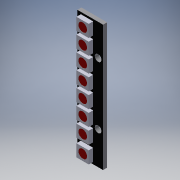
# Autodesk Inventor part: Neopixel_Stick
Saved by Autodesk Inventor 2016 (Build 200138000, 138)
## iProperties
Created: 2018-09-26
Part Number: Neopixel_Stick
Material: Generic
Document SubType Name: Modeling
Designer: Student
Density: 1 g/cm^3
Appearance: Default
Author: Student
Autodesk Inventor part; units mm, degrees
ref_plane "YZ Plane" through (0, 0, 0) normal (1, 0, 0) x (0, 1, 0)
ref_plane "XZ Plane" through (0, 0, 0) normal (0, 1, 0) x (-1, 0, 0)
ref_plane "XY Plane" through (0, 0, 0) normal (0, 0, 1) x (1, 0, 0)
sketch "Sketch1" plane through (0, 0, 0) normal (0, 0, 1) x (1, 0, 0)
  line L0 (0, 0) -> (10.414, 0)
  line L1 (10.414, 0) -> (10.414, 50.8)
  line L2 (10.414, 50.8) -> (0, 50.8)
  line L3 (0, 50.8) -> (0, 0)
  dimension "d0" = 10.414
  dimension "d1" = 50.8
  constraints: 8 end point, 2 parallel, 1 horizontal, 1 perpendicular
  measures "d0" distance of L2.end L1.end
  measures "d1" distance of L1.end L0.end
extrude "Extrusion1" add sketch "Sketch1" along normal blind 1.651
sketch "Sketch2" plane through (0, 0, 1.651) normal (0, 0, 1) x (1, 0, 0)
  line L0 (0, 0) -> (10.414, 0) projected
  line L1 (5.207, 0) -> (3.937, 0)
  line L2 (3.937, 0) -> (3.937, 3.302)
  circle A0 centre (3.937, 3.302) radius 1.778
  line L3 (10.414, 50.8) -> (0, 50.8) projected
  line L4 (5.207, 50.8) -> (3.937, 50.8)
  line L5 (3.937, 50.8) -> (3.937, 47.498)
  circle A1 centre (3.937, 47.498) radius 1.778
  line L6 (3.937, 47.498) -> (3.937, 41.275)
  line L7 (3.937, 41.275) -> (3.937, 35.052)
  line L8 (3.937, 35.052) -> (3.937, 28.829)
  line L9 (3.937, 28.829) -> (3.937, 22.606)
  line L10 (3.937, 22.606) -> (3.937, 16.383)
  line L11 (3.937, 16.383) -> (3.937, 10.16)
  line L12 (3.937, 10.16) -> (3.937, 3.302)
  circle A2 centre (3.937, 10.16) radius 1.778
  circle A3 centre (3.937, 16.383) radius 1.778
  circle A4 centre (3.937, 22.606) radius 1.778
  circle A5 centre (3.937, 28.829) radius 1.778
  circle A6 centre (3.937, 35.052) radius 1.778
  circle A7 centre (3.937, 41.275) radius 1.778
  line L13 (1.4605, 45.0215) -> (6.4135, 45.0215)
  line L14 (6.4135, 45.0215) -> (6.4135, 49.9745)
  line L15 (6.4135, 49.9745) -> (1.4605, 49.9745)
  line L16 (1.4605, 49.9745) -> (1.4605, 45.0215)
  line L17 (1.4605, 45.0215) -> (6.4135, 49.9745) construction
  line L18 (6.4135, 45.0215) -> (1.4605, 49.9745) construction
  line L19 (1.4605, 38.7985) -> (6.4135, 38.7985)
  line L20 (6.4135, 38.7985) -> (6.4135, 43.7515)
  line L21 (6.4135, 43.7515) -> (1.4605, 43.7515)
  line L22 (1.4605, 43.7515) -> (1.4605, 38.7985)
  line L23 (1.4605, 38.7985) -> (6.4135, 43.7515) construction
  line L24 (6.4135, 38.7985) -> (1.4605, 43.7515) construction
  line L25 (1.4605, 32.5755) -> (6.4135, 32.5755)
  line L26 (6.4135, 32.5755) -> (6.4135, 37.5285)
  line L27 (6.4135, 37.5285) -> (1.4605, 37.5285)
  line L28 (1.4605, 37.5285) -> (1.4605, 32.5755)
  line L29 (1.4605, 32.5755) -> (6.4135, 37.5285) construction
  line L30 (6.4135, 32.5755) -> (1.4605, 37.5285) construction
  line L31 (1.4605, 26.3525) -> (6.4135, 26.3525)
  line L32 (6.4135, 26.3525) -> (6.4135, 31.3055)
  line L33 (6.4135, 31.3055) -> (1.4605, 31.3055)
  line L34 (1.4605, 31.3055) -> (1.4605, 26.3525)
  line L35 (1.4605, 26.3525) -> (6.4135, 31.3055) construction
  line L36 (6.4135, 26.3525) -> (1.4605, 31.3055) construction
  line L37 (1.4605, 20.1295) -> (6.4135, 20.1295)
  line L38 (6.4135, 20.1295) -> (6.4135, 25.0825)
  line L39 (6.4135, 25.0825) -> (1.4605, 25.0825)
  line L40 (1.4605, 25.0825) -> (1.4605, 20.1295)
  line L41 (1.4605, 20.1295) -> (6.4135, 25.0825) construction
  line L42 (6.4135, 20.1295) -> (1.4605, 25.0825) construction
  line L43 (1.4605, 13.9065) -> (6.4135, 13.9065)
  line L44 (6.4135, 13.9065) -> (6.4135, 18.8595)
  line L45 (6.4135, 18.8595) -> (1.4605, 18.8595)
  line L46 (1.4605, 18.8595) -> (1.4605, 13.9065)
  line L47 (1.4605, 13.9065) -> (6.4135, 18.8595) construction
  line L48 (6.4135, 13.9065) -> (1.4605, 18.8595) construction
  line L49 (1.4605, 7.6835) -> (6.4135, 7.6835)
  line L50 (6.4135, 7.6835) -> (6.4135, 12.6365)
  line L51 (6.4135, 12.6365) -> (1.4605, 12.6365)
  line L52 (1.4605, 12.6365) -> (1.4605, 7.6835)
  line L53 (1.4605, 7.6835) -> (6.4135, 12.6365) construction
  line L54 (6.4135, 7.6835) -> (1.4605, 12.6365) construction
  line L55 (1.4605, 0.8255) -> (6.4135, 0.8255)
  line L56 (6.4135, 0.8255) -> (6.4135, 5.7785)
  line L57 (6.4135, 5.7785) -> (1.4605, 5.7785)
  line L58 (1.4605, 5.7785) -> (1.4605, 0.8255)
  line L59 (1.4605, 0.8255) -> (6.4135, 5.7785) construction
  line L60 (6.4135, 0.8255) -> (1.4605, 5.7785) construction
  dimension "d4" = 1.27
  dimension "d5" = 3.302
  dimension "d6" = 3.556
  dimension "d7" = 3.302
  dimension "d8" = 3.556
  dimension "d9" = 6.223
  dimension "d10" = 6.223
  dimension "d11" = 6.223
  dimension "d12" = 6.223
  dimension "d13" = 6.223
  dimension "d14" = 6.223
  dimension "d15" = 3.556
  dimension "d16" = 3.556
  dimension "d17" = 3.556
  dimension "d18" = 3.556
  dimension "d19" = 3.556
  dimension "d20" = 3.556
  dimension "d21" = 4.953
  dimension "d22" = 4.953
  dimension "d23" = 4.953
  dimension "d24" = 4.953
  dimension "d25" = 4.953
  dimension "d26" = 4.953
  dimension "d27" = 4.953
  dimension "d28" = 4.953
  dimension "d29" = 4.953
  dimension "d30" = 4.953
  dimension "d31" = 4.953
  dimension "d32" = 4.953
  constraints: 118 end point, 18 midpoint, 16 parallel, 11 point on line, 10 perpendicular, 8 centre point, 8 coincident, 8 horizontal, 1 collinear, 1 vertical
  measures "d4" distance of L1.start L1.end
  measures "d5" distance of L1.end L2.end
  measures "d6" diameter of A0
  measures "d7" distance of L4.end L5.end
  measures "d8" diameter of A1
  measures "d9" distance of L6.start L6.end
  measures "d10" distance of L6.end L7.end
  measures "d11" distance of L7.end L8.end
  measures "d12" distance of L8.end L9.end
  measures "d13" distance of L9.end L10.end
  measures "d14" distance of L10.end L11.end
  measures "d15" diameter of A2
  measures "d16" diameter of A3
  measures "d17" diameter of A4
  measures "d18" diameter of A5
  measures "d19" diameter of A6
  measures "d20" diameter of A7
  measures "d21" distance of L15.end L14.end
  measures "d22" distance of L14.end L13.end
  measures "d23" distance of L21.end L20.end
  measures "d24" distance of L20.end L19.end
  measures "d25" distance of L27.end L26.end
  measures "d26" distance of L26.end L25.end
  measures "d27" distance of L33.end L32.end
  measures "d28" distance of L32.end L31.end
  measures "d29" distance of L38.end L37.end
  measures "d30" distance of L44.end L43.end
  measures "d31" distance of L50.end L49.end
  measures "d32" distance of L56.end L55.end
extrude "Extrusion2" add sketch "Sketch2" along normal blind 1.778 contours L55 L58 L57 L12 A0 L2 | L13 L16 L15 L5 A1 L6 | L6 A1 L5 L15 L14 L13 | L19 L22 L21 L6 A7 L7 | L7 A7 L6 L21 L20 L19 | L25 L28 L27 L7 A6 L8 | L8 A6 L7 L27 L26 L25 | L31 L34 L33 L8 A5 L9 | L9 A5 L8 L33 L32 L31 | L37 L40 L39 L9 A4 L10 | L10 A4 L9 L39 L38 L37 | L43 L46 L45 L10 A3 L11 | L11 A3 L10 L45 L44 L43 | L49 L52 L51 L11 A2 L12 | L12 A2 L11 L51 L50 L49 | L2 A0 L12 L57 L56 L55
sketch "Sketch3" plane through (0, 0, 1.651) normal (0, 0, 1) x (1, 0, 0)
  circle A0 centre (3.937, 3.302) radius 1.778 projected
  circle A1 centre (3.937, 3.302) radius 1.778
  circle A2 centre (3.937, 10.16) radius 1.778 projected
  circle A3 centre (3.937, 10.16) radius 1.778
  circle A4 centre (3.937, 16.383) radius 1.778 projected
  circle A5 centre (3.937, 16.383) radius 1.778
  circle A6 centre (3.937, 22.606) radius 1.778 projected
  circle A7 centre (3.937, 22.606) radius 1.778
  circle A8 centre (3.937, 28.829) radius 1.778 projected
  circle A9 centre (3.937, 28.829) radius 1.778
  circle A10 centre (3.937, 35.052) radius 1.778 projected
  circle A11 centre (3.937, 35.052) radius 1.778
  circle A12 centre (3.937, 41.275) radius 1.778 projected
  circle A13 centre (3.937, 41.275) radius 1.778
  circle A14 centre (3.937, 47.498) radius 1.778 projected
  circle A15 centre (3.937, 47.498) radius 1.778
  point P0 (0, 0)
  constraints: 8 centre point, 8 coincident
extrude "Extrusion3" add sketch "Sketch3" along normal blind 1.651
sketch "Sketch4" plane through (0, 0, 1.651) normal (0, 0, 1) x (1, 0, 0)
  line L0 (1.4605, 12.6365) -> (6.4135, 12.6365) projected
  line L1 (6.4135, 13.9065) -> (6.4135, 18.8595) projected
  line L2 (6.4135, 12.6365) -> (6.4135, 13.9065)
  line L3 (6.4135, 13.9065) -> (6.4135, 13.2715)
  line L4 (10.414, 0) -> (10.414, 50.8) projected
  line L5 (10.414, 13.2715) -> (6.4135, 13.2715)
  circle A0 centre (8.4138, 13.2715) radius 1.3335
  line L6 (1.4605, 37.5285) -> (6.4135, 37.5285) projected
  line L7 (6.4135, 38.7985) -> (6.4135, 37.5285)
  line L8 (6.4135, 38.1635) -> (10.414, 38.1635)
  circle A1 centre (8.4138, 38.1635) radius 1.3335
  point P0 (0, 0)
  constraints: 10 end point, 4 midpoint, 2 centre point, 2 perpendicular, 2 point on line, 2 vertical
extrude "Extrusion4" cut sketch "Sketch4" against normal blind 1.651
body "Solid1"
